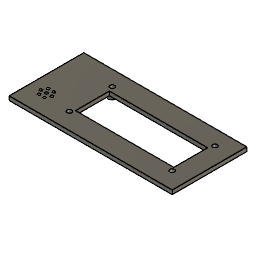
Front_panel_v05 (Autodesk Fusion 360 design; units mm, degrees)
part number: 2026-08-01-20-36-51-163
Autodesk Fusion 360 part; units mm, degrees
sketch "Sketch1" plane through (0, 0, 0) normal (0, 0, 1) x (1, 0, 0)
  line L0 (60, -27.5) -> (-60, -27.5)
  line L1 (-60, -27.5) -> (-60, 27.5)
  line L2 (-60, 27.5) -> (60, 27.5)
  line L3 (60, 27.5) -> (60, -27.5)
  line L4 (60, -27.5) -> (-60, 27.5) construction
  line L5 (-60, -27.5) -> (60, 27.5) construction
  dimension "d1" = 120
  dimension "d2" = 55
  constraint horizontal L0
  constraint perpendicular L0 L1
  constraint parallel L0 L2
  constraint parallel L1 L3
  constraint coincident L4 origin
  constraint coincident L5 origin
  measures "d1" distance of L1.end L2.end
  measures "d2" distance of L0.end L1.end
extrude "Extrude1" add sketch "Sketch1" along normal blind 3
sketch "Sketch2" plane through (0, 0, 3) normal (0, 0, 1) x (-1, 0, 0)
  line L0 (-60, -27.5) -> (60, -27.5)
  line L1 (60, -27.5) -> (60, 27.5)
  line L2 (60, 27.5) -> (-60, 27.5)
  line L3 (-60, 27.5) -> (-60, -27.5)
  line L4 (26.1, 12.4) -> (-46.1, 12.4)
  line L5 (-46.1, 12.4) -> (-46.1, -12.4)
  line L6 (-46.1, -12.4) -> (26.1, -12.4)
  line L7 (26.1, -12.4) -> (26.1, 12.4)
  line L8 (26.1, 12.4) -> (-46.1, -12.4) construction
  line L9 (-46.1, 12.4) -> (26.1, -12.4) construction
  point P0 (-10, 0)
  dimension "d5" = 72.2
  dimension "d6" = 24.8
  constraint horizontal L4
  constraint perpendicular L4 L5
  constraint parallel L4 L6
  constraint parallel L5 L7
  constraint coincident L8 P0
  constraint coincident L9 P0
  measures "d5" distance of L5.end L6.end
  measures "d6" distance of L4.end L5.end
extrude "Extrude2" cut sketch "Sketch2" against normal through all contours L4 L5 L6 L7
sketch "Sketch3" plane through (0, 0, 3) normal (0, 0, 1) x (-1, 0, 0)
  line L0 (26.1, -12.4) -> (-46.1, -12.4)
  line L1 (-46.1, -12.4) -> (-46.1, 12.4)
  line L2 (-46.1, 12.4) -> (26.1, 12.4)
  line L3 (26.1, 12.4) -> (26.1, -12.4)
  line L4 (-60, -27.5) -> (60, -27.5)
  line L5 (60, -27.5) -> (60, 27.5)
  line L6 (60, 27.5) -> (-60, 27.5)
  line L7 (-60, 27.5) -> (-60, -27.5)
  circle A0 centre (27.9, -16.35) radius 1.7
  circle A1 centre (-47.66, -16.35) radius 1.7
  circle A2 centre (27.9, 15.18) radius 1.7
  circle A3 centre (-47.66, 15.18) radius 1.7
  dimension "d9" = 3.4
  dimension "d10" = 27.9
  dimension "d11" = 16.35
  dimension "d14" = 75.56
  dimension "d15" = -31.53
  measures "d9" diameter of A0
  measures "d10" horizontal distance of origin A0.centre
  measures "d11" vertical distance of origin A0.centre
extrude "Extrude3" cut sketch "Sketch3" against normal through all contours A0 | A1 | A2 | A3
sketch "Sketch5" plane through (0, 0, 3) normal (0, 0, 1) x (-1, 0, 0)
  circle A0 centre (-47.66, 15.18) radius 1.7
  circle A1 centre (27.9, 15.18) radius 1.7
  circle A2 centre (27.9, -16.35) radius 1.7
  circle A3 centre (-47.66, -16.35) radius 1.7
  line L0 (26.1, -12.4) -> (-46.1, -12.4)
  line L1 (-46.1, -12.4) -> (-46.1, 12.4)
  line L2 (-46.1, 12.4) -> (26.1, 12.4)
  line L3 (26.1, 12.4) -> (26.1, -12.4)
  line L4 (-60, -27.5) -> (60, -27.5)
  line L5 (60, -27.5) -> (60, 27.5)
  line L6 (60, 27.5) -> (-60, 27.5)
  line L7 (-60, 27.5) -> (-60, -27.5)
  line L8 (56.1021, -14.9687) -> (33, -15) construction
  line L9 (33, -15) -> (33.013, -24.5594) construction
  line L10 (33.013, -24.5594) -> (56.1151, -24.5281) construction
  line L11 (56.1151, -24.5281) -> (56.1021, -14.9687) construction
  dimension "d24" = 3.5
sketch "Sketch6" plane through (0, 0, 3) normal (0, 0, 1) x (-1, 0, 0)
  line L0 (-60, -27.5) -> (60, -27.5)
  line L1 (60, -27.5) -> (60, 27.5)
  line L2 (60, 27.5) -> (-60, 27.5)
  line L3 (-60, 27.5) -> (-60, -27.5)
  line L4 (26.1, -12.4) -> (-46.1, -12.4)
  line L5 (-46.1, -12.4) -> (-46.1, 12.4)
  line L6 (-46.1, 12.4) -> (26.1, 12.4)
  line L7 (26.1, 12.4) -> (26.1, -12.4)
  circle A0 centre (-47.66, -16.35) radius 1.7
  circle A1 centre (27.9, -16.35) radius 1.7
  circle A2 centre (27.9, 15.18) radius 1.7
  circle A3 centre (-47.66, 15.18) radius 1.7
  circle A4 centre (48, 12) radius 1
  circle A5 centre (44, 12) radius 1
  circle A6 centre (46, 8.5359) radius 1
  circle A7 centre (50, 8.5359) radius 1
  circle A8 centre (52, 12) radius 1
  circle A9 centre (50, 15.4641) radius 1
  circle A10 centre (46, 15.4641) radius 1
  dimension "d29" = 2
  dimension "d30" = 48
  dimension "d31" = 12
  dimension "d32" = 2
  dimension "d33" = 4
  dimension "d35" = 360
  measures "d29" diameter of A4
  measures "d30" horizontal distance of origin A4.centre
  measures "d31" vertical distance of origin A4.centre
  measures "d32" diameter of A5
  measures "d33" distance of A4.centre A5.centre
extrude "Extrude6" cut sketch "Sketch6" against normal through all contours A4 | A5 | A6 | A7 | A8 | A9 | A10
sketch "Sketch7" plane through (0, 0, 0) normal (0, 0, 1) x (1, 0, 0)
  arc A0 (-40.7716, -10) -> (-40.7716, -14) centre (-48, -12) ccw
  arc A1 (-42.4493, -10) -> (-42.4493, -14) centre (-48, -12) ccw
  line L0 (-40.7716, -10) -> (-42.4493, -10)
  line L1 (-40.7716, -14) -> (-42.4493, -14)
  dimension "d37" = 11.8
  dimension "d38" = 48
  dimension "d39" = 12
  dimension "d40" = 15
  dimension "d41" = 2
  dimension "d42" = 2
  constraint concentric A0 A1
  constraint horizontal L0
  constraint horizontal L1
  measures "d37" diameter of A1
  measures "d38" horizontal distance of origin A0.centre
  measures "d39" vertical distance of origin A0.centre
  measures "d40" diameter of A0
  measures "d41" distance of A0.centre L0
  measures "d42" distance of A0.centre L1
extrude "Extrude7" add sketch "Sketch7" against normal blind 5.5
sketch "Sketch8" plane through (0, 0, 0) normal (0, 0, -1) x (1, 0, 0)
  circle A0 centre (-46, 15.4641) radius 1
  circle A1 centre (-48, 12) radius 1
  circle A2 centre (-50, 15.4641) radius 1
  circle A3 centre (-44, 12) radius 1
  circle A4 centre (-50, 8.5359) radius 1
  circle A5 centre (-52, 12) radius 1
  circle A6 centre (-46, 8.5359) radius 1
  line L0 (-60, -27.5) -> (60, -27.5)
  line L1 (60, -27.5) -> (60, 27.5)
  line L2 (60, 27.5) -> (-60, 27.5)
  line L3 (-60, 27.5) -> (-60, -27.5)
  line L4 (46.1, -12.4) -> (-26.1, -12.4)
  line L5 (-26.1, -12.4) -> (-26.1, 12.4)
  line L6 (-26.1, 12.4) -> (46.1, 12.4)
  line L7 (46.1, 12.4) -> (46.1, -12.4)
  circle A7 centre (47.66, -16.35) radius 1.7
  circle A8 centre (-27.9, -16.35) radius 1.7
  circle A9 centre (-27.9, 15.18) radius 1.7
  circle A10 centre (47.66, 15.18) radius 1.7
  line L8 (-40.7716, 14) -> (-42.4493, 14)
  arc A11 (-42.4493, 14) -> (-42.4493, 10) centre (-48, 12) ccw
  line L9 (-42.4493, 10) -> (-40.7716, 10)
  arc A12 (-40.7716, 14) -> (-40.7716, 10) centre (-48, 12) ccw
  circle A13 centre (47.66, -16.35) radius 1.7
  circle A14 centre (-27.9, -16.35) radius 1.7
  circle A15 centre (-27.9, 15.18) radius 1.7
  circle A16 centre (47.66, 15.18) radius 1.7
  circle A17 centre (47.66, -16.35) radius 3.5
  circle A18 centre (-27.9, -16.35) radius 3.5
  arc A19 (46.1, 12.0469) -> (45.5336, 12.4) centre (47.66, 15.18) ccw
  arc A20 (-25.7736, 12.4) -> (-26.1, 12.1783) centre (-27.9, 15.18) ccw
  point P0 (46.1, 12.4)
  point P1 (46.1, -12.4)
  point P2 (-26.1, -12.4)
  point P3 (-26.1, 12.4)
  dimension "d45" = 7
  dimension "d46" = 7
  dimension "d47" = 7
  dimension "d48" = 7
  constraint concentric A13 A17
  constraint concentric A14 A18
  constraint concentric A16 A19
  constraint concentric A15 A20
  constraint coincident L6 A19.end
  constraint coincident L7 A19.start
  constraint coincident L5 A20.end
  constraint coincident L6 A20.start
  measures "d45" diameter of A17
  measures "d46" diameter of A18
  measures "d47" diameter of A19
  measures "d48" diameter of A20
extrude "Extrude8" add sketch "Sketch8" along normal blind 3 contours L6 L7 A19 | L5 L6 A20 | A17 | A18
equation "d25 = 'Teo larmklocka'"
